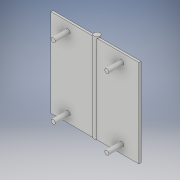
# Autodesk Inventor part: Hinge
Saved by Autodesk Inventor 2019 (Build 230136000, 136)
## iProperties
Created: 2018-10-04
Part Number: Hinge
Material: Generic
Document SubType Name: Modeling
Designer: abhay
Density: 1 g/cm^3
Appearance: Default
Author: abhay
Autodesk Inventor part; units mm, degrees
ref_plane "YZ Plane" through (0, 0, 0) normal (1, 0, 0) x (0, 1, 0)
ref_plane "XZ Plane" through (0, 0, 0) normal (0, 1, 0) x (-1, 0, 0)
ref_plane "XY Plane" through (0, 0, 0) normal (0, 0, 1) x (1, 0, 0)
sketch "Sketch1" plane through (0, 0, 0) normal (0, 0, 1) x (1, 0, 0)
  line L0 (-44.45, -44.323) -> (44.45, -44.323)
  line L1 (44.45, -44.323) -> (44.45, 44.323)
  line L2 (44.45, 44.323) -> (-44.45, 44.323)
  line L3 (-44.45, 44.323) -> (-44.45, -44.323)
  line L4 (-44.45, -44.323) -> (44.45, 44.323) construction
  line L5 (44.45, -44.323) -> (-44.45, 44.323) construction
  point P0 (0, 0)
  dimension "d0" = 88.9
  dimension "d1" = 88.646
  constraints: 12 end point, 2 midpoint, 2 parallel, 1 horizontal, 1 perpendicular
  measures "d0" distance of L2.end L1.end
  measures "d1" distance of L1.end L0.end
extrude "Extrusion1" add sketch "Sketch1" along normal blind 2.159
sketch "Sketch3" plane through (-44.45, 44.323, 0) normal (0, 1, 0) x (1, 0, 0)
  circle A0 centre (44.45, 0) radius 2.9972
  dimension "d4" = 5.9944
  constraints: 1 centre point, 1 coincident
  measures "d4" diameter of A0
extrude "Extrusion2" add sketch "Sketch3" along normal blind 1.27 and the other way blind 88.773
sketch "Sketch4" plane through (0, 0, 2.159) normal (0, 0, 1) x (1, 0, 0)
  circle A0 centre (-27.1018, 35.7124) radius 2.1828
  line L0 (-44.45, 44.323) -> (-44.45, -44.323) projected
  line L1 (-2.0789, 44.323) -> (-44.45, 44.323) projected
  line L2 (-44.45, 0) -> (0, 0)
  circle A1 centre (-27.1018, -35.7124) radius 2.1828
  line L3 (-2.9972, -44.45) -> (2.9972, -44.45) projected
  line L4 (0, -44.45) -> (0, 45.593)
  line L5 (2.9972, 45.593) -> (-2.9972, 45.593) projected
  circle A2 centre (27.1018, 35.7124) radius 2.1828
  circle A3 centre (27.1018, -35.7124) radius 2.1828
  dimension "d9" = 17.3482
  dimension "d10" = 4.3656
  dimension "d11" = 8.6106
  constraints: 4 centre point, 4 end point, 3 midpoint, 3 symmetric about line, 1 horizontal, 3 other
  measures "d9" distance from line of L0 A0.centre
  measures "d10" diameter of A0
  measures "d11" distance from line of L1 A0.centre
extrude "Extrusion3" add sketch "Sketch4" along normal blind 15 and the other way blind 5
body "Solid1"
